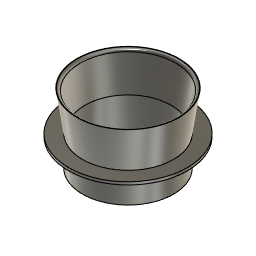
Food_funnel (Autodesk Fusion 360 design; units mm, degrees)
Autodesk Fusion 360 part; units mm, degrees
note: some values were not read from the file. Set by a fixed rule: which face or edge a step refers to.
sketch "Sketch1" plane through (0, 0, 0) normal (0, 0, 1) x (1, 0, 0)
  circle A0 centre (0, 0) radius 30.5
  circle A1 centre (0, 0) radius 32.5
  dimension "d7" = 61
  dimension "d8" = 65
  constraint coincident A0.centre A1.centre
  measures "d7" diameter of A0
  measures "d8" diameter of A1
extrude "Extrude1" add sketch "Sketch1" along normal blind 19.5
ref_plane "WorkPlane1" through (0, 0, 19.5) normal (0, 0, 1) x (1, 0, 0)
sketch "Sketch2" plane through (0, 0, 19.5) normal (0, 0, 1) x (1, 0, 0)
  circle A0 centre (0, 0) radius 42.5
  circle A1 centre (0, 0) radius 30.5
  dimension "d13" = 85
  dimension "d15" = 61
  constraint coincident A0.centre A1.centre
  measures "d13" diameter of A0
  measures "d15" diameter of A1
extrude "Extrude2" add sketch "Sketch2" along normal blind 2
ref_plane "WorkPlane2" through (0, 0, 49.5) normal (0, 0, 1) x (1, 0, 0)
sketch "Sketch3" plane through (0, 0, 49.5) normal (0, 0, 1) x (1, 0, 0)
  circle A0 centre (0, 0) radius 34.5
  circle A1 centre (0, 0) radius 36.5
  dimension "d19" = 69
  dimension "d20" = 73
  constraint coincident A0.centre A1.centre
  constraint concentric A0 A1
  measures "d19" diameter of A0
  measures "d20" diameter of A1
ref_plane "WorkPlane3" through (0, 0, 21.5) normal (0, 0, 1) x (1, 0, 0)
sketch "Sketch4" plane through (0, 0, 21.5) normal (0, 0, 1) x (1, 0, 0)
  circle A0 centre (0, 0) radius 30.5
  circle A1 centre (0, 0) radius 32.5
  dimension "d22" = 61
  dimension "d23" = 65
  constraint coincident A0.centre A1.centre
  measures "d22" diameter of A0
  measures "d23" diameter of A1
loft "Loft1" add profiles "Sketch4", "Sketch3" section 1 section 2
shell "Shell1" thickness 2 removed faces 1 at (-3.2479, -15.4478, 49.5)
extrude "Extrude3" cut 1 faces at (-2.282, 9.0945, 23.5) along direction (0, 0, -1) up to surface (23.5 mm away)
fillet "Fillet1" radius 2 1 edges at (-32.1464, 12.4684, 49.5)
equation "Bottom_outter_dia = 65 mm"
equation "Bottom_inner_dia = 61 mm"
equation "bottom_height = 19.5 mm"
equation "Top_outter_dia = 73 mm"
equation "Top_inner_dia = 69 mm"
equation "Top_height = 30 mm"
equation "d7 = Bottom_inner_dia"
equation "d8 = Bottom_outter_dia"
equation "d9 = bottom_height"
equation "d11 = bottom_height"
equation "flange_dia = 85 mm"
equation "d13 = flange_dia"
equation "Flange_height = 2 mm"
equation "d15 = Bottom_inner_dia"
equation "d16 = Flange_height"
equation "d18 = Top_height + bottom_height"
equation "d19 = Top_inner_dia"
equation "d20 = Top_outter_dia"
equation "d22 = Bottom_inner_dia"
equation "d23 = Bottom_outter_dia"
